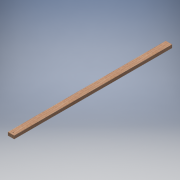
# Autodesk Inventor part: 1x2 Longitudinal
Saved by Autodesk Inventor 2019 (Build 230136000, 136)
## iProperties
Created: 2020-12-30
Part Number: 1x2 Longitudinal
Material: Wood (Birch)
Document SubType Name: Modeling
Designer: John
Density: 0.55 g/cm^3
Appearance: Birch - Natural Polished
Author: John
Autodesk Inventor part; units mm, degrees
ref_plane "YZ Plane" through (0, 0, 0) normal (1, 0, 0) x (0, 1, 0)
ref_plane "XZ Plane" through (0, 0, 0) normal (0, 1, 0) x (-1, 0, 0)
ref_plane "XY Plane" through (0, 0, 0) normal (0, 0, 1) x (1, 0, 0)
sketch "Sketch1" plane through (0, 0, 0) normal (0, 0, 1) x (1, 0, 0)
  line L0 (-19.05, -9.525) -> (19.05, -9.525)
  line L1 (19.05, -9.525) -> (19.05, 9.525)
  line L2 (19.05, 9.525) -> (-19.05, 9.525)
  line L3 (-19.05, 9.525) -> (-19.05, -9.525)
  line L4 (-19.05, -9.525) -> (19.05, 9.525) construction
  line L5 (19.05, -9.525) -> (-19.05, 9.525) construction
  point P0 (0, 0)
  dimension "d0" = 38.1
  dimension "d1" = 19.05
  constraints: 12 end point, 2 midpoint, 2 parallel, 1 horizontal, 1 perpendicular
  measures "d0" distance of L2.end L1.end
  measures "d1" distance of L1.end L0.end
extrude "Extrusion1" add sketch "Sketch1" along normal mid plane 959.0278
sketch "Sketch2" plane through (-19.05, -9.525, 479.5139) normal (0, -1, 0) x (1, 0, 0)
  circle A0 centre (19.05, -12.7508) radius 2.2225
  line L0 (0, 0) -> (38.1, 0) projected
  line L1 (0, 0) -> (0, -959.0278) projected
  point P0 (19.05, -479.5139)
  dimension "d4" = 4.445
  dimension "d5" = 12.7508
  dimension "d6" = 19.05
  constraints: 1 centre point
  measures "d4" diameter of A0
  measures "d5" distance from line of L0 A0.centre
  measures "d6" distance from line of L1 A0.centre
extrude "Extrusion2" cut sketch "Sketch2" against normal blind 25.4
sketch "Sketch3" plane through (-19.05, -9.525, 479.5139) normal (0, -1, 0) x (1, 0, 0)
  circle A0 centre (19.05, -12.7508) radius 2.2225 projected
  circle A1 centre (19.05, -12.7508) radius 4.1275
  point P0 (19.05, -479.5139)
  dimension "d9" = 8.255
  constraints: 1 centre point, 1 coincident
  measures "d9" diameter of A1
extrude "Extrusion3" cut sketch "Sketch3" against normal blind 12.7
mirror "Mirror1" about plane through (0, 0, 0) normal (0, 0, 1) of "Extrusion2", "Extrusion3"
body "Solid1"
